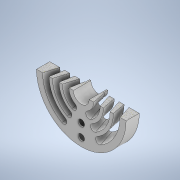
# Autodesk Inventor part: Мой ограничитель
Saved by Autodesk Inventor 2021 (Build 250183000, 183)
## iProperties
Created: 2020-11-07
Part Number: Мой ограничитель
Material: Типовые
Document SubType Name: Modeling
Designer: Тимоха
Density: 1 g/cm^3
Appearance: По умолчанию
Author: Тимоха
Autodesk Inventor part; units mm, degrees
ref_plane "YZ Plane" through (0, 0, 0) normal (1, 0, 0) x (0, 1, 0)
ref_plane "XZ Plane" through (0, 0, 0) normal (0, 1, 0) x (-1, 0, 0)
ref_plane "XY Plane" through (0, 0, 0) normal (0, 0, 1) x (1, 0, 0)
sketch "Эскиз1" plane through (0, 0, 0) normal (0, 0, 1) x (1, 0, 0)
  circle A0 centre (0, 0) radius 68
  dimension "d0" = 136
  constraints: 1 centre point, 1 coincident
  measures "d0" diameter of A0
extrude "Выдавливание1" add sketch "Эскиз1" along normal blind 20
sketch "Эскиз2" plane through (0, 0, 0) normal (0, 0, -1) x (-1, 0, 0)
  circle A0 centre (0, 0) radius 15
  dimension "d3" = 30
  constraints: 1 centre point, 1 coincident
  measures "d3" diameter of A0
extrude "Выдавливание2" add sketch "Эскиз2" along normal blind 6.5
sketch "Эскиз4" plane through (0, 0, 20) normal (0, 0, 1) x (1, 0, 0)
  circle A0 centre (0, 0) radius 15 projected
  circle A1 centre (0, 0) radius 68 projected
  circle A2 centre (0, 0) radius 20 projected
  arc A3 (9.375, 16.238) -> (14.375, 24.8982) centre (11.875, 20.5681) ccw
  arc A4 (17.0187, 29.1477) -> (22.0737, 37.7732) centre (19.6413, 33.4047) ccw
  arc A5 (24.375, 42.2187) -> (29.375, 50.879) centre (26.875, 46.5489) ccw
  arc A6 (9.375, 16.238) -> (-9.375, 16.238) centre (0, 0) ccw
  arc A7 (17.0187, 29.1477) -> (-17.1076, 29.0956) centre (0, 0) ccw
  arc A8 (24.375, 42.2187) -> (-24.375, 42.2187) centre (0, 0) ccw
  arc A9 (14.375, 24.8982) -> (-14.375, 24.8982) centre (0, 0) ccw
  arc A10 (22.276, 37.6542) -> (-22.175, 37.7138) centre (0, 0) ccw
  arc A11 (29.375, 50.879) -> (-29.375, 50.879) centre (0, 0) ccw
  arc A12 (-22.175, 37.7138) -> (-17.1076, 29.0956) centre (-19.6413, 33.4047) ccw
  arc A13 (-29.375, 50.879) -> (-24.375, 42.2187) centre (-26.875, 46.5489) ccw
  arc A14 (-14.375, 24.8982) -> (-9.375, 16.238) centre (-11.875, 20.5681) ccw
  arc A15 (-58.75, 0) -> (-29.375, -50.879) centre (0, 0) ccw
  arc A16 (-29.375, -50.879) -> (-24.375, -42.2187) centre (-26.875, -46.5489) ccw
  arc A17 (-48.75, 0) -> (-24.375, -42.2187) centre (0, 0) ccw
  arc A18 (-48.75, 0) -> (-58.75, 0) centre (-53.75, 0) ccw
  arc A19 (-33.752, 0.1647) -> (-43.7494, 0.2298) centre (-38.75, 0.3075) ccw
  arc A20 (-33.752, 0.1647) -> (-16.6437, -29.3635) centre (0, 0) ccw
  arc A21 (-21.5737, -38.061) -> (-16.6437, -29.3635) centre (-19.1087, -33.7122) ccw
  arc A22 (-43.7475, 0.4645) -> (-21.5737, -38.061) centre (0, 0) ccw
  arc A23 (-28.75, 0) -> (-14.375, -24.8982) centre (0, 0) ccw
  arc A24 (-14.375, -24.8982) -> (-9.375, -16.238) centre (-11.875, -20.5681) ccw
  arc A25 (-18.75, 0) -> (-9.375, -16.238) centre (0, 0) ccw
  arc A26 (-18.75, 0) -> (-28.75, 0) centre (-23.75, 0) ccw
  arc A27 (29.375, -50.879) -> (58.75, 0) centre (0, 0) ccw
  arc A28 (58.75, 0) -> (48.75, 0) centre (53.75, 0) ccw
  arc A29 (24.375, -42.2187) -> (48.75, 0) centre (0, 0) ccw
  arc A30 (24.375, -42.2187) -> (29.375, -50.879) centre (26.875, -46.5489) ccw
  arc A31 (16.7333, -29.3125) -> (21.6757, -38.003) centre (19.1087, -33.7122) ccw
  arc A32 (16.7333, -29.3125) -> (33.7514, 0.2678) centre (0, 0) ccw
  arc A33 (43.7486, 0.3472) -> (33.7514, 0.2678) centre (38.75, 0.3075) ccw
  arc A34 (21.4715, -38.1187) -> (43.7486, 0.3472) centre (0, 0) ccw
  arc A35 (14.375, -24.8982) -> (28.75, 0) centre (0, 0) ccw
  arc A36 (28.75, 0) -> (18.75, 0) centre (23.75, 0) ccw
  arc A37 (9.375, -16.238) -> (18.75, 0) centre (0, 0) ccw
  arc A38 (9.375, -16.238) -> (14.375, -24.8982) centre (11.875, -20.5681) ccw
  dimension "d18" = 10
  dimension "d19" = 10
  dimension "d20" = 10
  dimension "d22" = 87.5
  dimension "d26" = 360
  constraints: 78 point on circle, 36 centre point, 22 coincident, 7 tangent, 112 other
  measures "d18" diameter of A3
  measures "d19" diameter of A4
  measures "d20" diameter of A5
  measures "d22" diameter of A10
sketch "Эскиз3" plane through (0, 0, 0) normal (0, 0, -1) x (-1, 0, 0)
  arc A0 (7.5, 12.9904) -> (11.25, 19.4856) centre (9.375, 16.238) ccw
  arc A1 (15, 25.9808) -> (18.7172, 32.4984) centre (17.1085, 29.0971) ccw
  arc A2 (22.5, 38.9711) -> (26.25, 45.4663) centre (24.375, 42.2187) ccw
  arc A3 (-11.25, 19.4856) -> (-7.5, 12.9904) centre (-9.375, 16.238) ccw
  arc A4 (-18.6989, 32.5076) -> (-14.9489, 26.0124) centre (-17.0902, 29.1062) ccw
  arc A5 (-26.25, 45.4663) -> (-22.5, 38.9711) centre (-24.375, 42.2187) ccw
  arc A6 (22.5, 38.9711) -> (-22.5, 38.9711) centre (0, 0) ccw
  arc A7 (26.25, 45.4663) -> (-26.25, 45.4663) centre (0, 0) ccw
  arc A8 (19.2986, 32.1566) -> (-19.2646, 32.1769) centre (0, 0) ccw
  arc A9 (15.4104, 25.7394) -> (-15.4104, 25.7394) centre (0, 0) ccw
  arc A10 (11.25, 19.4856) -> (-11.25, 19.4856) centre (0, 0) ccw
  arc A11 (7.5, -12.9904) -> (11.25, -19.4856) centre (9.375, -16.238) ccw
  arc A12 (11.25, -19.4856) -> (22.5, 0) centre (0, 0) ccw
  arc A13 (22.5, 0) -> (15, 0) centre (18.75, 0) ccw
  arc A14 (37.5019, -0.06) -> (30.0019, -0.06) centre (33.7519, 0.2474) ccw
  arc A15 (52.5, 0) -> (45, 0) centre (48.75, 0) ccw
  arc A16 (14.5858, -26.2155) -> (29.9962, 0.4761) centre (0, 0) ccw
  arc A17 (15, -25.9808) -> (18.7859, -32.4588) centre (16.6446, -29.3649) ccw
  arc A18 (18.1991, -32.7913) -> (37.4983, 0.5951) centre (0, 0) ccw
  arc A19 (22.5, -38.9711) -> (45, 0) centre (0, 0) ccw
  arc A20 (22.5, -38.9711) -> (26.25, -45.4663) centre (24.375, -42.2187) ccw
  arc A21 (26.25, -45.4663) -> (52.5, 0) centre (0, 0) ccw
  arc A22 (-15, 0) -> (-22.5, 0) centre (-18.75, 0) ccw
  arc A23 (-22.5, 0) -> (-11.25, -19.4856) centre (0, 0) ccw
  arc A24 (-11.25, -19.4856) -> (-7.5, -12.9904) centre (-9.375, -16.238) ccw
  arc A25 (-18.8029, -32.4475) -> (-15.0529, -25.9523) centre (-16.6616, -29.3537) ccw
  arc A26 (-26.25, -45.4663) -> (-22.5, -38.9711) centre (-24.375, -42.2187) ccw
  arc A27 (-29.9962, 0.4761) -> (-14.5858, -26.2155) centre (0, 0) ccw
  arc A28 (-30, 0) -> (-37.503, -0.0397) centre (-33.753, 0.2678) ccw
  arc A29 (-37.4977, 0.6348) -> (-18.2338, -32.7721) centre (0, 0) ccw
  arc A30 (-45, 0) -> (-22.5, -38.9711) centre (0, 0) ccw
  arc A31 (-45, 0) -> (-52.5, 0) centre (-48.75, 0) ccw
  arc A32 (-52.5, 0) -> (-26.25, -45.4663) centre (0, 0) ccw
  arc A33 (7.5, -12.9904) -> (15, 0) centre (0, 0) ccw
  arc A34 (-15, 0) -> (-7.5, -12.9904) centre (0, 0) ccw
  arc A35 (7.5, 12.9904) -> (-7.5, 12.9904) centre (0, 0) ccw
  dimension "d12" = 3.75
  dimension "d13" = 3.7626
  dimension "d16" = 360
  dimension "d60" = 15
  dimension "d61" = 30
  dimension "d62" = 45
  constraints: 91 point on circle, 36 centre point, 20 coincident, 122 other
  measures "d12" radius of A0
  measures "d13" radius of A1
  measures "d60" radius of A35
  measures "d61" radius of A9
  measures "d62" radius of A6
loft "Лофт1" cut profiles "Эскиз4", "Эскиз3" contours A2 A38 A37 A36 | A2 A36 A35 A38 / A34 A24 A23 A22
loft "Лофт2" cut profiles "Эскиз3", "Эскиз4" contours A29 A28 A27 A25 / A32 A33 A34 A31
loft "Лофт3" cut profiles "Эскиз4", "Эскиз3" contours A30 A29 A28 A27 / A32 A31 A30 A26
pattern_circular "Круговой массив1" count 3 over 360 about axis through (0, 0, -10) along (0, 0, 1) of "Лофт3", "Лофт2", "Лофт1"
sketch "Эскиз5" plane through (0, 0, 0) normal (0, 0, -1) x (-1, 0, 0)
  line L0 (0, 0) -> (68, 0)
  circle A0 centre (0, 0) radius 68 projected
  line L1 (0, 0) -> (66.8973, 38.6232)
  circle A1 centre (31.8886, 18.4109) radius 8
  circle A2 centre (48.3265, 27.9013) radius 8
  dimension "d45" = 30
  dimension "d46" = 16
  dimension "d47" = 16
  constraints: 4 end point, 2 centre point, 2 point on line, 1 horizontal, 1 horizontal alignment, 1 other
  measures "d45" angle of L1 L0
  measures "d46" diameter of A1
  measures "d47" diameter of A2
extrude "Выдавливание3" cut sketch "Эскиз5" against normal blind 18 contours A1 L1 | L1 A1 | A2 L1 | L1 A2
sketch "Эскиз6" plane through (-31.8886, 18.4109, 18) normal (0, 0, -1) x (-1, 0, 0)
  circle A0 centre (0, 0) radius 5
  circle A1 centre (16.4379, 9.4904) radius 8 projected
  circle A2 centre (16.4379, 9.4904) radius 5
  point P0 (-31.8886, -18.4109)
  dimension "d50" = 10
  dimension "d51" = 10
  constraints: 2 centre point, 1 coincident
  measures "d50" diameter of A0
  measures "d51" diameter of A2
extrude "Выдавливание4" cut sketch "Эскиз6" against normal blind 18 contours A0 | A2
pattern_circular "Круговой массив2" count 3 over 360 about axis through (0, 0, -10) along (0, 0, 1) of "Выдавливание4", "Выдавливание3"
sketch "Эскиз7" plane through (0, 0, -6.5) normal (0, 0, -1) x (-1, 0, 0)
  circle A0 centre (0, 0) radius 12
  dimension "d57" = 24
  constraints: 1 centre point, 1 coincident
  measures "d57" diameter of A0
extrude "Выдавливание5" cut sketch "Эскиз7" against normal blind 28.5
sketch "Эскиз8" plane through (0, 0, -6.5) normal (0, 0, -1) x (-1, 0, 0)
  circle A0 centre (0, 0) radius 14
  circle A1 centre (0, 0) radius 15 projected
  dimension "d64" = 28
  constraints: 1 centre point, 1 coincident
  measures "d64" diameter of A0
extrude "Выдавливание6" cut sketch "Эскиз8" against normal blind 6.5
